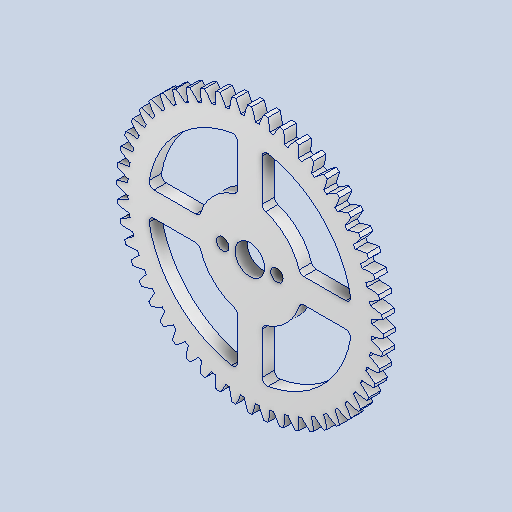
# Autodesk Inventor part: 平歯車1
Saved by Autodesk Inventor 2025.2 (Build 292293000, 293)
## iProperties
CustomPartVersion: 1
Created: 2025-05-14
Part Number: 平歯車1
Material: アルミニウム 6061
Document SubType Name: Modeling
Designer: haruy
Categories: <?xml version="1.0" encoding="UTF-16"?> <MemberInstance><Categories><FamilyTemplate><FamilyTemplateParameter ValueType="xs:double" Id="1" ObjectReferenceKey="da_z" ObjectType="kUserParameterObject"/><FamilyTemplateParameter ValueType="xs:double" Id="2" ObjectReferenceKey="da_b" ObjectType="kUserParameterObject"/><FamilyTemplateParameter ValueType="xs:double" Id="3" ObjectReferenceKey="da_beta" ObjectType="kUserParameterObject"/><FamilyTemplateParameter ValueType="xs:double" Id="4" ObjectReferenceKey="da_da" ObjectType="kUserParameterObject"/><FamilyTemplateParameter ValueType="xs:double" Id="5" ObjectReferenceKey="da_aw" ObjectType="kUserParameterObject"/><FamilyTemplateParameter ValueType="xs:string" Id="6" ObjectReferenceKey="EAIAABAAAACIAQAAAAAAAIAAAAAAAAAA" ObjectType="83910656" SubObjectId="SurfaceGeometry"/></FamilyTemplate><ParamToTemplateMap><ParamToTemplate CategoryParameter="//CategoryParameter[@InternalName='046C89C9-8512-4d59-83FE-43B91F4F132A']" TemplateParameter="1"/><ParamToTemplate CategoryParameter="//CategoryParameter[@InternalName='2552DF32-E462-4b46-AEBF-C6C7768E72AC']" TemplateParameter="2"/><ParamToTemplate CategoryParameter="//CategoryParameter[@InternalName='C9EE641D-15FC-4fae-A226-E94C4372FDD7']" TemplateParameter="3"/><ParamToTemplate><ParamToTemplate CategoryParameter="//CategoryParameter[@InternalName='00B6519A-459B-49c7-AD84-2E56D39A5744']" ConstantValue="0.000000"/></ParamToTemplate><ParamToTemplate><ParamToTemplate CategoryParameter="//CategoryParameter[@InternalName='04B31F0E-C7A6-4894-AA32-9629BEFACF47']" ConstantValue="1.000000"/></ParamToTemplate><ParamToTemplate><ParamToTemplate CategoryParameter="//CategoryParameter[@InternalName='43CBEC2E-7847-49e7-A936-2F7889FCB2D9']" ConstantValue="0.250000"/></ParamToTemplate><ParamToTemplate><ParamToTemplate CategoryParameter="//CategoryParameter[@InternalName='B1EFC894-105D-4ebd-86BF-FA20ED196853']" ConstantValue="0.350000"/></ParamToTemplate><ParamToTemplate><ParamToTemplate CategoryParameter="//CategoryParameter[@InternalName='51175063-3D10-4879-93E8-6246FE8B403D']" ConstantValue="2060000000.000000"/></ParamToTemplate><ParamToTemplate><ParamToTemplate CategoryParameter="//CategoryParameter[@InternalName='A3A52E27-4454-46a9-B0BD-C932399B70AF']" ConstantValue="0.300000"/></ParamToTemplate><ParamToTemplate><ParamToTemplate CategoryParameter="//CategoryParameter[@InternalName='91B76062-C214-41d9-B1B9-14D2AB99603D']" ConstantValue="0.200000"/></ParamToTemplate><ParamToTemplate><ParamToTemplate CategoryParameter="//CategoryParameter[@InternalName='374E806E-8B8A-4dda-A9AA-1039D6500AD2']" ConstantValue="5.000000"/></ParamToTemplate><ParamToTemplate><ParamToTemplate CategoryParameter="//CategoryParameter[@InternalName='2D373A89-B862-43d6-8D0B-0CBF12AB9F6C']" ConstantValue="0.349066"/></ParamToTemplate><ParamToTemplate CategoryParameter="//CategoryParameter[@InternalName='37777632-D6A2-4fac-9D53-DB8ACD95C989']" TemplateParameter="4"/><ParamToTemplate CategoryParameter="//CategoryParameter[@InternalName='FD1017F1-B727-4f7e-9707-0F86F1FF9423']" TemplateParameter="5"/><ParamToTemplate><ParamToTemplate CategoryParameter="//CategoryParameter[@InternalName='9E1B4470-B2D3-4ff1-B813-535BB4CDF51A']" ConstantValue="3520000.000000"/></ParamToTemplate><ParamToTemplate><ParamToTemplate CategoryParameter="//CategoryParameter[@InternalName='F8452263-BFF6-458c-9FB1-07C4B99E95CD']" ConstantValue="11400000.000000"/></ParamToTemplate><ParamToTemplate><ParamToTemplate CategoryParameter="//CategoryParameter[@InternalName='3E3BB259-FD49-497f-8171-6EBC954A3479']" ConstantValue="2.000000"/></ParamToTemplate><ParamToTemplate CategoryParameter="//CategoryParameter[@InternalName='27C3BAF2-7550-4e4b-AE2C-0DB134B7D9B7']" TemplateParameter="6"/></ParamToTemplateMap><Category DisplayName="Gear" InternalName="DC85795E-93AB-48d5-8EEE-5A27447B64BD" Mnemonic="Gear"><CategoryParameter DisplayName="z" InternalName="046C89C9-8512-4d59-83FE-43B91F4F132A" Mnemonic="z"/><CategoryParameter DisplayName="b" InternalName="2552DF32-E462-4b46-AEBF-C6C7768E72AC" Mnemonic="b"/><CategoryParameter DisplayName="||b|" InternalName="C9EE641D-15FC-4fae-A226-E94C4372FDD7" Mnemonic="beta"/><CategoryParameter DisplayName="x" InternalName="00B6519A-459B-49c7-AD84-2E56D39A5744" Mnemonic="x"/><CategoryParameter DisplayName="a*" InternalName="04B31F0E-C7A6-4894-AA32-9629BEFACF47" Mnemonic="a"/><CategoryParameter DisplayName="c*" InternalName="43CBEC2E-7847-49e7-A936-2F7889FCB2D9" Mnemonic="c"/><CategoryParameter DisplayName="r|.f|*" InternalName="B1EFC894-105D-4ebd-86BF-FA20ED196853" Mnemonic="rf"/><CategoryParameter DisplayName="E" InternalName="51175063-3D10-4879-93E8-6246FE8B403D" Mnemonic="E"/><CategoryParameter DisplayName="||m|" InternalName="A3A52E27-4454-46a9-B0BD-C932399B70AF" Mnemonic="mi"/><Category DisplayName="SpurGear" InternalName="26C5A22E-A91E-4dfd-A3B3-23CCAFAE1764" Mnemonic="SpurGear"><CategoryParameter DisplayName="m" InternalName="91B76062-C214-41d9-B1B9-14D2AB99603D" Mnemonic="m"/><CategoryParameter DisplayName="P" InternalName="374E806E-8B8A-4dda-A9AA-1039D6500AD2" Mnemonic="PP"/><CategoryParameter DisplayName="||a|" InternalName="2D373A89-B862-43d6-8D0B-0CBF12AB9F6C" Mnemonic="alpha"/><CategoryParameter DisplayName="d|.a|" InternalName="37777632-D6A2-4fac-9D53-DB8ACD95C989" Mnemonic="da"/><CategoryParameter DisplayName="a|.w|" InternalName="FD1017F1-B727-4f7e-9707-0F86F1FF9423" Mnemonic="aw"/><CategoryParameter DisplayName="||s||.Flim|" InternalName="9E1B4470-B2D3-4ff1-B813-535BB4CDF51A" Mnemonic="sFlim"/><CategoryParameter DisplayName="||s||.Hlim|" InternalName="F8452263-BFF6-458c-9FB1-07C4B99E95CD" Mnemonic="sHlim"/><CategoryParameter DisplayName="タイプ" InternalName="3E3BB259-FD49-497f-8171-6EBC954A3479" Mnemonic="type"/><CategoryParameter DisplayName="PitchDiameter" InternalName="27C3BAF2-7550-4e4b-AE2C-0DB134B7D9B7" Mnemonic="IDS_PITCHDIAM"/></Category></Category></Categories></MemberInstance>
Density: 2.7 g/cm^3
Appearance: アルミニウム - フラット
Author: haruy
Autodesk Inventor part; units mm, degrees
sketch "Sketch1" plane through (0, 0, 0) normal (0, 0, 1) x (1, 0, 0)
  circle A0 centre (0, 0) radius 54
  dimension "d0" = 108
  constraints: 1 centre point
  measures "d0" diameter of A0
extrude "Extrusion1" add sketch "Sketch1" along normal blind 5
ref_plane "Work Plane2" through (0, 0, 2.5) normal (0, 0, 1) x (1, 0, 0)
sketch "Sketch2" plane through (0, 0, 0) normal (0, 0, -1) x (-1, 0, 0)
  circle A0 centre (0, 0) radius 54 projected
  circle A1 centre (0, 0) radius 52
  dimension "d3" = 104
  constraints: 1 centre point, 1 coincident
  measures "d3" diameter of A1
surface extrude "ピッチ円直径" sketch "Sketch2" against normal through all shown no curves A1
ref_plane "Work Plane8" through (0, 0, 0) normal (0.9981756, 0.0603785, 0) x (0, 0, 1)
ref_plane "Work Plane9" through (0, 0, 0) normal (1, 0, 0) x (0, 1, 0)
spur gear teeth "平歯車" teeth 52 pitch diameter 104 tip diameter 108 root diameter 99 face width 5 start plane through (0, 0, 0) normal (0, 0, -1) x (-1, 0, 0)
sketch "スケッチ3" plane through (0, 0, 5) normal (0, 0, 1) x (1, 0, 0)
  circle A0 centre (0, 0) radius 6
  circle A1 centre (0, 0) radius 11
  circle A2 centre (-11, 0) radius 2.5
  circle A3 centre (11, 0) radius 2.5
  circle A4 centre (0, 0) radius 49.5
  circle A5 centre (0, 0) radius 21
  circle A6 centre (0, 0) radius 41.5
  line L0 (-5, 41.1977) -> (-5, 20.3961)
  line L1 (0, 0) -> (0, 49.5)
  line L2 (5, 41.1977) -> (5, 20.3961)
  line L3 (-41.1977, -5) -> (-20.3961, -5)
  line L4 (-41.1977, 5) -> (-20.3961, 5)
  line L5 (5, -41.1977) -> (5, -20.3961)
  line L6 (-5, -41.1977) -> (-5, -20.3961)
  line L7 (41.1977, 5) -> (20.3961, 5)
  line L8 (41.1977, -5) -> (20.3961, -5)
  point P0 (-49.4492, 2.2421)
  dimension "d50" = 22
  dimension "d56" = 10
  dimension "d49" = 12
  dimension "d51" = 5
  dimension "d54" = 360
  dimension "d57" = 8
  dimension "d58" = 5
  dimension "d61" = 360
  constraints: 18 end point, 4 centre point, 3 coincident, 2 point on circle, 2 symmetric about line, 1 horizontal alignment, 1 parallel, 1 vertical, 38 other
  measures "d49" diameter of A0
  measures "d51" diameter of A2
  measures "d58" distance between parallel lines of L1 L0
extrude "押し出し2" cut sketch "スケッチ3" against normal blind 10 contours A0 | A1 A3 | A1 A3 | A2 A1 | A1 A2 | A5 L2 A6 L7 | L8 A6 L5 A5 | L6 A6 L3 A5 | A5 L4 A6 L0
fillet "フィレット1" radius 2 16 edges at (-41.1977, -5, 2.5) (-20.3961, -5, 2.5) (-5, -20.3961, 2.5) (-5, -41.1977, 2.5) (5, -20.3961, 2.5) (5, -41.1977, 2.5) (41.1977, -5, 2.5) (20.3961, -5, 2.5) (20.3961, 5, 2.5) (41.1977, 5, 2.5) (5, 20.3961, 2.5) (5, 41.1977, 2.5) (-5, 41.1977, 2.5) (-5, 20.3961, 2.5) (-20.3961, 5, 2.5) (-41.1977, 5, 2.5)
sketch "スケッチ5" plane through (0, 0, 5) normal (0, 0, 1) x (1, 0, 0)
  line L0 (5, -38.8748) -> (5, -21.9089) projected
  arc A0 (6.3913, -20.0038) -> (5, -21.9089) centre (7, -21.9089) ccw projected
  arc A1 (6.3913, -20.0038) -> (20.0038, -6.3913) centre (0, 0) ccw projected
  arc A2 (21.9089, -5) -> (20.0038, -6.3913) centre (21.9089, -7) ccw projected
  line L1 (21.9089, -5) -> (38.8748, -5) projected
  arc A3 (40.8431, -7.3544) -> (38.8748, -5) centre (38.8748, -7) ccw projected
  arc A4 (7.3544, -40.8431) -> (40.8431, -7.3544) centre (0, 0) ccw projected
  arc A5 (5, -38.8748) -> (7.3544, -40.8431) centre (7, -38.8748) ccw projected
  circle A6 centre (11, 0) radius 2.5 projected
  line L2 (5, 21.9089) -> (5, 38.8748) projected
  arc A7 (7.3544, 40.8431) -> (5, 38.8748) centre (7, 38.8748) ccw projected
  arc A8 (40.8431, 7.3544) -> (7.3544, 40.8431) centre (0, 0) ccw projected
  arc A9 (38.8748, 5) -> (40.8431, 7.3544) centre (38.8748, 7) ccw projected
  line L3 (38.8748, 5) -> (21.9089, 5) projected
  arc A10 (20.0038, 6.3913) -> (21.9089, 5) centre (21.9089, 7) ccw projected
  arc A11 (20.0038, 6.3913) -> (6.3913, 20.0038) centre (0, 0) ccw projected
  arc A12 (5, 21.9089) -> (6.3913, 20.0038) centre (7, 21.9089) ccw projected
  line L4 (-38.8748, -5) -> (-21.9089, -5) projected
  arc A13 (-20.0038, -6.3913) -> (-21.9089, -5) centre (-21.9089, -7) ccw projected
  arc A14 (-20.0038, -6.3913) -> (-6.3913, -20.0038) centre (0, 0) ccw projected
  arc A15 (-5, -21.9089) -> (-6.3913, -20.0038) centre (-7, -21.9089) ccw projected
  line L5 (-5, -21.9089) -> (-5, -38.8748) projected
  arc A16 (-7.3544, -40.8431) -> (-5, -38.8748) centre (-7, -38.8748) ccw projected
  arc A17 (-40.8431, -7.3544) -> (-7.3544, -40.8431) centre (0, 0) ccw projected
  arc A18 (-38.8748, -5) -> (-40.8431, -7.3544) centre (-38.8748, -7) ccw projected
  circle A19 centre (-11, 0) radius 2.5 projected
  circle A20 centre (0, 0) radius 6 projected
  line L6 (-5, 38.8748) -> (-5, 21.9089) projected
  arc A21 (-6.3913, 20.0038) -> (-5, 21.9089) centre (-7, 21.9089) ccw projected
  arc A22 (-6.3913, 20.0038) -> (-20.0038, 6.3913) centre (0, 0) ccw projected
  arc A23 (-21.9089, 5) -> (-20.0038, 6.3913) centre (-21.9089, 7) ccw projected
  line L7 (-21.9089, 5) -> (-38.8748, 5) projected
  arc A24 (-40.8431, 7.3544) -> (-38.8748, 5) centre (-38.8748, 7) ccw projected
  arc A25 (-7.3544, 40.8431) -> (-40.8431, 7.3544) centre (0, 0) ccw projected
  arc A26 (-5, 38.8748) -> (-7.3544, 40.8431) centre (-7, 38.8748) ccw projected
  arc A27 (-7.3179, 53.5019) -> (-8.1862, 48.8184) centre (15.9886, 46.7583) ccw projected
  arc A28 (-8.1862, 48.8184) -> (-9.657, 48.5489) centre (0, 0) ccw projected
  arc A29 (-9.657, 48.5489) -> (-12.1297, 52.6201) centre (-31.5303, 38.0502) ccw projected
  arc A30 (-12.1297, 52.6201) -> (-13.7134, 52.2297) centre (0, 0) ccw projected
  arc A31 (-13.7134, 52.2297) -> (-14.011, 47.4757) centre (10.2359, 48.3446) ccw projected
  arc A32 (-14.011, 47.4757) -> (-15.4385, 47.0309) centre (0, 0) ccw projected
  arc A33 (-15.4385, 47.0309) -> (-18.3839, 50.7743) centre (-35.8868, 33.9722) ccw projected
  arc A34 (-18.3839, 50.7743) -> (-19.9091, 50.1959) centre (0, 0) ccw projected
  arc A35 (-19.9091, 50.1959) -> (-19.6314, 45.4407) centre (4.334, 49.2259) ccw projected
  arc A36 (-19.6314, 45.4407) -> (-20.9949, 44.8271) centre (0, 0) ccw projected
  arc A37 (-20.9949, 44.8271) -> (-24.37, 48.1882) centre (-39.7201, 29.3988) ccw projected
  arc A38 (-24.37, 48.1882) -> (-25.8143, 47.4302) centre (0, 0) ccw projected
  arc A39 (-25.8143, 47.4302) -> (-24.9655, 42.7431) centre (-1.6312, 49.3894) ccw projected
  arc A40 (-24.9655, 42.7431) -> (-26.2451, 41.9696) centre (0, 0) ccw projected
  arc A41 (-26.2451, 41.9696) -> (-30.0008, 44.8994) centre (-42.9741, 24.3967) ccw projected
  arc A42 (-30.0008, 44.8994) -> (-31.3432, 43.9728) centre (0, 0) ccw projected
  arc A43 (-31.3432, 43.9728) -> (-29.9356, 39.4222) centre (-7.5725, 48.8327) ccw projected
  arc A44 (-29.9356, 39.4222) -> (-31.1126, 38.5001) centre (0, 0) ccw projected
  arc A45 (-31.1126, 38.5001) -> (-35.1941, 40.9558) centre (-45.6015, 19.0389) ccw projected
  arc A46 (-35.1941, 40.9558) -> (-36.415, 39.8741) centre (0, 0) ccw projected
  arc A47 (-36.415, 39.8741) -> (-34.4692, 35.5264) centre (-13.4034, 47.5639) ccw projected
  arc A48 (-34.4692, 35.5264) -> (-35.5264, 34.4692) centre (0, 0) ccw projected
  arc A49 (-35.5264, 34.4692) -> (-39.8741, 36.415) centre (-47.5639, 13.4034) ccw projected
  arc A50 (-39.8741, 36.415) -> (-40.9558, 35.1941) centre (0, 0) ccw projected
  arc A51 (-40.9558, 35.1941) -> (-38.5001, 31.1126) centre (-19.0389, 45.6015) ccw projected
  arc A52 (-38.5001, 31.1126) -> (-39.4222, 29.9356) centre (0, 0) ccw projected
  arc A53 (-39.4222, 29.9356) -> (-43.9728, 31.3432) centre (-48.8327, 7.5725) ccw projected
  arc A54 (-43.9728, 31.3432) -> (-44.8994, 30.0008) centre (0, 0) ccw projected
  arc A55 (-44.8994, 30.0008) -> (-41.9696, 26.2451) centre (-24.3967, 42.9741) ccw projected
  arc A56 (-41.9696, 26.2451) -> (-42.7431, 24.9655) centre (0, 0) ccw projected
  arc A57 (-42.7431, 24.9655) -> (-47.4302, 25.8143) centre (-49.3894, 1.6312) ccw projected
  arc A58 (-47.4302, 25.8143) -> (-48.1882, 24.37) centre (0, 0) ccw projected
  arc A59 (-48.1882, 24.37) -> (-44.8271, 20.9949) centre (-29.3988, 39.7201) ccw projected
  arc A60 (-44.8271, 20.9949) -> (-45.4407, 19.6314) centre (0, 0) ccw projected
  arc A61 (-45.4407, 19.6314) -> (-50.1959, 19.9091) centre (-49.2259, -4.334) ccw projected
  arc A62 (-50.1959, 19.9091) -> (-50.7743, 18.3839) centre (0, 0) ccw projected
  arc A63 (-50.7743, 18.3839) -> (-47.0309, 15.4385) centre (-33.9722, 35.8868) ccw projected
  arc A64 (-47.0309, 15.4385) -> (-47.4757, 14.011) centre (0, 0) ccw projected
  arc A65 (-47.4757, 14.011) -> (-52.2297, 13.7134) centre (-48.3446, -10.2359) ccw projected
  arc A66 (-52.2297, 13.7134) -> (-52.6201, 12.1297) centre (0, 0) ccw projected
  arc A67 (-52.6201, 12.1297) -> (-48.5489, 9.657) centre (-38.0502, 31.5303) ccw projected
  arc A68 (-48.5489, 9.657) -> (-48.8184, 8.1862) centre (0, 0) ccw projected
  arc A69 (-48.8184, 8.1862) -> (-53.5019, 7.3179) centre (-46.7583, -15.9886) ccw projected
  arc A70 (-53.5019, 7.3179) -> (-53.6985, 5.6986) centre (0, 0) ccw projected
  arc A71 (-53.6985, 5.6986) -> (-49.3589, 3.7346) centre (-41.5733, 26.7139) ccw projected
  arc A72 (-49.3589, 3.7346) -> (-49.4492, 2.2421) centre (0, 0) ccw projected
  arc A73 (-49.4492, 2.2421) -> (-53.9938, 0.8156) centre (-44.4902, -21.5081) ccw projected
  arc A74 (-53.9938, 0.8156) -> (-53.9938, -0.8156) centre (0, 0) ccw projected
  arc A75 (-53.9938, -0.8156) -> (-49.4492, -2.2421) centre (-44.4902, 21.5081) ccw projected
  arc A76 (-49.4492, -2.2421) -> (-49.3589, -3.7346) centre (0, 0) ccw projected
  arc A77 (-49.3589, -3.7346) -> (-53.6985, -5.6986) centre (-41.5733, -26.7139) ccw projected
  arc A78 (-53.6985, -5.6986) -> (-53.5019, -7.3179) centre (0, 0) ccw projected
  arc A79 (-53.5019, -7.3179) -> (-48.8184, -8.1862) centre (-46.7583, 15.9886) ccw projected
  arc A80 (-48.8184, -8.1862) -> (-48.5489, -9.657) centre (0, 0) ccw projected
  arc A81 (-48.5489, -9.657) -> (-52.6201, -12.1297) centre (-38.0502, -31.5303) ccw projected
  arc A82 (-52.6201, -12.1297) -> (-52.2297, -13.7134) centre (0, 0) ccw projected
  arc A83 (-52.2297, -13.7134) -> (-47.4757, -14.011) centre (-48.3446, 10.2359) ccw projected
  arc A84 (-47.4757, -14.011) -> (-47.0309, -15.4385) centre (0, 0) ccw projected
  arc A85 (-47.0309, -15.4385) -> (-50.7743, -18.3839) centre (-33.9722, -35.8868) ccw projected
  arc A86 (-50.7743, -18.3839) -> (-50.1959, -19.9091) centre (0, 0) ccw projected
  arc A87 (-50.1959, -19.9091) -> (-45.4407, -19.6314) centre (-49.2259, 4.334) ccw projected
  arc A88 (-45.4407, -19.6314) -> (-44.8271, -20.9949) centre (0, 0) ccw projected
  arc A89 (-44.8271, -20.9949) -> (-48.1882, -24.37) centre (-29.3988, -39.7201) ccw projected
  arc A90 (-48.1882, -24.37) -> (-47.4302, -25.8143) centre (0, 0) ccw projected
  arc A91 (-47.4302, -25.8143) -> (-42.7431, -24.9655) centre (-49.3894, -1.6312) ccw projected
  arc A92 (-42.7431, -24.9655) -> (-41.9696, -26.2451) centre (0, 0) ccw projected
  arc A93 (-41.9696, -26.2451) -> (-44.8994, -30.0008) centre (-24.3967, -42.9741) ccw projected
  arc A94 (-44.8994, -30.0008) -> (-43.9728, -31.3432) centre (0, 0) ccw projected
  arc A95 (-43.9728, -31.3432) -> (-39.4222, -29.9356) centre (-48.8327, -7.5725) ccw projected
  arc A96 (-39.4222, -29.9356) -> (-38.5001, -31.1126) centre (0, 0) ccw projected
  arc A97 (-38.5001, -31.1126) -> (-40.9558, -35.1941) centre (-19.0389, -45.6015) ccw projected
  arc A98 (-40.9558, -35.1941) -> (-39.8741, -36.415) centre (0, 0) ccw projected
  arc A99 (-39.8741, -36.415) -> (-35.5264, -34.4692) centre (-47.5639, -13.4034) ccw projected
  arc A100 (-35.5264, -34.4692) -> (-34.4692, -35.5264) centre (0, 0) ccw projected
  arc A101 (-34.4692, -35.5264) -> (-36.415, -39.8741) centre (-13.4034, -47.5639) ccw projected
  arc A102 (-36.415, -39.8741) -> (-35.1941, -40.9558) centre (0, 0) ccw projected
  arc A103 (-35.1941, -40.9558) -> (-31.1126, -38.5001) centre (-45.6015, -19.0389) ccw projected
  arc A104 (-31.1126, -38.5001) -> (-29.9356, -39.4222) centre (0, 0) ccw projected
  arc A105 (-29.9356, -39.4222) -> (-31.3432, -43.9728) centre (-7.5725, -48.8327) ccw projected
  arc A106 (-31.3432, -43.9728) -> (-30.0008, -44.8994) centre (0, 0) ccw projected
  arc A107 (-30.0008, -44.8994) -> (-26.2451, -41.9696) centre (-42.9741, -24.3967) ccw projected
  arc A108 (-26.2451, -41.9696) -> (-24.9655, -42.7431) centre (0, 0) ccw projected
  arc A109 (-24.9655, -42.7431) -> (-25.8143, -47.4302) centre (-1.6312, -49.3894) ccw projected
  arc A110 (-25.8143, -47.4302) -> (-24.37, -48.1882) centre (0, 0) ccw projected
  arc A111 (-24.37, -48.1882) -> (-20.9949, -44.8271) centre (-39.7201, -29.3988) ccw projected
  arc A112 (-20.9949, -44.8271) -> (-19.6314, -45.4407) centre (0, 0) ccw projected
  arc A113 (-19.6314, -45.4407) -> (-19.9091, -50.1959) centre (4.334, -49.2259) ccw projected
  arc A114 (-19.9091, -50.1959) -> (-18.3839, -50.7743) centre (0, 0) ccw projected
  arc A115 (-18.3839, -50.7743) -> (-15.4385, -47.0309) centre (-35.8868, -33.9722) ccw projected
  arc A116 (-15.4385, -47.0309) -> (-14.011, -47.4757) centre (0, 0) ccw projected
  arc A117 (-14.011, -47.4757) -> (-13.7134, -52.2297) centre (10.2359, -48.3446) ccw projected
  arc A118 (-13.7134, -52.2297) -> (-12.1297, -52.6201) centre (0, 0) ccw projected
  arc A119 (-12.1297, -52.6201) -> (-9.657, -48.5489) centre (-31.5303, -38.0502) ccw projected
  arc A120 (-9.657, -48.5489) -> (-8.1862, -48.8184) centre (0, 0) ccw projected
  arc A121 (-8.1862, -48.8184) -> (-7.3179, -53.5019) centre (15.9886, -46.7583) ccw projected
  arc A122 (-7.3179, -53.5019) -> (-5.6986, -53.6985) centre (0, 0) ccw projected
  arc A123 (-5.6986, -53.6985) -> (-3.7346, -49.3589) centre (-26.7139, -41.5733) ccw projected
  arc A124 (-3.7346, -49.3589) -> (-2.2421, -49.4492) centre (0, 0) ccw projected
  arc A125 (-2.2421, -49.4492) -> (-0.8156, -53.9938) centre (21.5081, -44.4902) ccw projected
  arc A126 (-0.8156, -53.9938) -> (0.8156, -53.9938) centre (0, 0) ccw projected
  arc A127 (0.8156, -53.9938) -> (2.2421, -49.4492) centre (-21.5081, -44.4902) ccw projected
  arc A128 (2.2421, -49.4492) -> (3.7346, -49.3589) centre (0, 0) ccw projected
  arc A129 (3.7346, -49.3589) -> (5.6986, -53.6985) centre (26.7139, -41.5733) ccw projected
  arc A130 (5.6986, -53.6985) -> (7.3179, -53.5019) centre (0, 0) ccw projected
  arc A131 (7.3179, -53.5019) -> (8.1862, -48.8184) centre (-15.9886, -46.7583) ccw projected
  arc A132 (8.1862, -48.8184) -> (9.657, -48.5489) centre (0, 0) ccw projected
  arc A133 (9.657, -48.5489) -> (12.1297, -52.6201) centre (31.5303, -38.0502) ccw projected
  arc A134 (12.1297, -52.6201) -> (13.7134, -52.2297) centre (0, 0) ccw projected
  arc A135 (13.7134, -52.2297) -> (14.011, -47.4757) centre (-10.2359, -48.3446) ccw projected
  arc A136 (14.011, -47.4757) -> (15.4385, -47.0309) centre (0, 0) ccw projected
  arc A137 (15.4385, -47.0309) -> (18.3839, -50.7743) centre (35.8868, -33.9722) ccw projected
  arc A138 (18.3839, -50.7743) -> (19.9091, -50.1959) centre (0, 0) ccw projected
  arc A139 (19.9091, -50.1959) -> (19.6314, -45.4407) centre (-4.334, -49.2259) ccw projected
  arc A140 (19.6314, -45.4407) -> (20.9949, -44.8271) centre (0, 0) ccw projected
  arc A141 (20.9949, -44.8271) -> (24.37, -48.1882) centre (39.7201, -29.3988) ccw projected
  arc A142 (24.37, -48.1882) -> (25.8143, -47.4302) centre (0, 0) ccw projected
  arc A143 (25.8143, -47.4302) -> (24.9655, -42.7431) centre (1.6312, -49.3894) ccw projected
  arc A144 (24.9655, -42.7431) -> (26.2451, -41.9696) centre (0, 0) ccw projected
  arc A145 (26.2451, -41.9696) -> (30.0008, -44.8994) centre (42.9741, -24.3967) ccw projected
  arc A146 (30.0008, -44.8994) -> (31.3432, -43.9728) centre (0, 0) ccw projected
  arc A147 (31.3432, -43.9728) -> (29.9356, -39.4222) centre (7.5725, -48.8327) ccw projected
  arc A148 (29.9356, -39.4222) -> (31.1126, -38.5001) centre (0, 0) ccw projected
  arc A149 (31.1126, -38.5001) -> (35.1941, -40.9558) centre (45.6015, -19.0389) ccw projected
  arc A150 (35.1941, -40.9558) -> (36.415, -39.8741) centre (0, 0) ccw projected
  arc A151 (36.415, -39.8741) -> (34.4692, -35.5264) centre (13.4034, -47.5639) ccw projected
  arc A152 (34.4692, -35.5264) -> (35.5264, -34.4692) centre (0, 0) ccw projected
  arc A153 (35.5264, -34.4692) -> (39.8741, -36.415) centre (47.5639, -13.4034) ccw projected
  arc A154 (39.8741, -36.415) -> (40.9558, -35.1941) centre (0, 0) ccw projected
  arc A155 (40.9558, -35.1941) -> (38.5001, -31.1126) centre (19.0389, -45.6015) ccw projected
  arc A156 (38.5001, -31.1126) -> (39.4222, -29.9356) centre (0, 0) ccw projected
  arc A157 (39.4222, -29.9356) -> (43.9728, -31.3432) centre (48.8327, -7.5725) ccw projected
  arc A158 (43.9728, -31.3432) -> (44.8994, -30.0008) centre (0, 0) ccw projected
  arc A159 (44.8994, -30.0008) -> (41.9696, -26.2451) centre (24.3967, -42.9741) ccw projected
  arc A160 (41.9696, -26.2451) -> (42.7431, -24.9655) centre (0, 0) ccw projected
  arc A161 (42.7431, -24.9655) -> (47.4302, -25.8143) centre (49.3894, -1.6312) ccw projected
  arc A162 (47.4302, -25.8143) -> (48.1882, -24.37) centre (0, 0) ccw projected
  arc A163 (48.1882, -24.37) -> (44.8271, -20.9949) centre (29.3988, -39.7201) ccw projected
  arc A164 (44.8271, -20.9949) -> (45.4407, -19.6314) centre (0, 0) ccw projected
  arc A165 (45.4407, -19.6314) -> (50.1959, -19.9091) centre (49.2259, 4.334) ccw projected
  arc A166 (50.1959, -19.9091) -> (50.7743, -18.3839) centre (0, 0) ccw projected
  arc A167 (50.7743, -18.3839) -> (47.0309, -15.4385) centre (33.9722, -35.8868) ccw projected
  arc A168 (47.0309, -15.4385) -> (47.4757, -14.011) centre (0, 0) ccw projected
  arc A169 (47.4757, -14.011) -> (52.2297, -13.7134) centre (48.3446, 10.2359) ccw projected
  arc A170 (52.2297, -13.7134) -> (52.6201, -12.1297) centre (0, 0) ccw projected
  arc A171 (52.6201, -12.1297) -> (48.5489, -9.657) centre (38.0502, -31.5303) ccw projected
  arc A172 (48.5489, -9.657) -> (48.8184, -8.1862) centre (0, 0) ccw projected
  arc A173 (48.8184, -8.1862) -> (53.5019, -7.3179) centre (46.7583, 15.9886) ccw projected
  arc A174 (53.5019, -7.3179) -> (53.6985, -5.6986) centre (0, 0) ccw projected
  arc A175 (53.6985, -5.6986) -> (49.3589, -3.7346) centre (41.5733, -26.7139) ccw projected
  arc A176 (49.3589, -3.7346) -> (49.4492, -2.2421) centre (0, 0) ccw projected
  arc A177 (49.4492, -2.2421) -> (53.9938, -0.8156) centre (44.4902, 21.5081) ccw projected
  arc A178 (53.9938, -0.8156) -> (53.9938, 0.8156) centre (0, 0) ccw projected
  arc A179 (53.9938, 0.8156) -> (49.4492, 2.2421) centre (44.4902, -21.5081) ccw projected
  arc A180 (49.4492, 2.2421) -> (49.3589, 3.7346) centre (0, 0) ccw projected
  arc A181 (49.3589, 3.7346) -> (53.6985, 5.6986) centre (41.5733, 26.7139) ccw projected
  arc A182 (53.6985, 5.6986) -> (53.5019, 7.3179) centre (0, 0) ccw projected
  arc A183 (53.5019, 7.3179) -> (48.8184, 8.1862) centre (46.7583, -15.9886) ccw projected
  arc A184 (48.8184, 8.1862) -> (48.5489, 9.657) centre (0, 0) ccw projected
  arc A185 (48.5489, 9.657) -> (52.6201, 12.1297) centre (38.0502, 31.5303) ccw projected
  arc A186 (52.6201, 12.1297) -> (52.2297, 13.7134) centre (0, 0) ccw projected
  arc A187 (52.2297, 13.7134) -> (47.4757, 14.011) centre (48.3446, -10.2359) ccw projected
  arc A188 (47.4757, 14.011) -> (47.0309, 15.4385) centre (0, 0) ccw projected
  arc A189 (47.0309, 15.4385) -> (50.7743, 18.3839) centre (33.9722, 35.8868) ccw projected
  arc A190 (50.7743, 18.3839) -> (50.1959, 19.9091) centre (0, 0) ccw projected
  arc A191 (50.1959, 19.9091) -> (45.4407, 19.6314) centre (49.2259, -4.334) ccw projected
  arc A192 (45.4407, 19.6314) -> (44.8271, 20.9949) centre (0, 0) ccw projected
  arc A193 (44.8271, 20.9949) -> (48.1882, 24.37) centre (29.3988, 39.7201) ccw projected
  arc A194 (48.1882, 24.37) -> (47.4302, 25.8143) centre (0, 0) ccw projected
  arc A195 (47.4302, 25.8143) -> (42.7431, 24.9655) centre (49.3894, 1.6312) ccw projected
  arc A196 (42.7431, 24.9655) -> (41.9696, 26.2451) centre (0, 0) ccw projected
  arc A197 (41.9696, 26.2451) -> (44.8994, 30.0008) centre (24.3967, 42.9741) ccw projected
  arc A198 (44.8994, 30.0008) -> (43.9728, 31.3432) centre (0, 0) ccw projected
  arc A199 (43.9728, 31.3432) -> (39.4222, 29.9356) centre (48.8327, 7.5725) ccw projected
  arc A200 (39.4222, 29.9356) -> (38.5001, 31.1126) centre (0, 0) ccw projected
  arc A201 (38.5001, 31.1126) -> (40.9558, 35.1941) centre (19.0389, 45.6015) ccw projected
  arc A202 (40.9558, 35.1941) -> (39.8741, 36.415) centre (0, 0) ccw projected
  arc A203 (39.8741, 36.415) -> (35.5264, 34.4692) centre (47.5639, 13.4034) ccw projected
  arc A204 (35.5264, 34.4692) -> (34.4692, 35.5264) centre (0, 0) ccw projected
  arc A205 (34.4692, 35.5264) -> (36.415, 39.8741) centre (13.4034, 47.5639) ccw projected
  arc A206 (36.415, 39.8741) -> (35.1941, 40.9558) centre (0, 0) ccw projected
  arc A207 (35.1941, 40.9558) -> (31.1126, 38.5001) centre (45.6015, 19.0389) ccw projected
  arc A208 (31.1126, 38.5001) -> (29.9356, 39.4222) centre (0, 0) ccw projected
  arc A209 (29.9356, 39.4222) -> (31.3432, 43.9728) centre (7.5725, 48.8327) ccw projected
  arc A210 (31.3432, 43.9728) -> (30.0008, 44.8994) centre (0, 0) ccw projected
  arc A211 (30.0008, 44.8994) -> (26.2451, 41.9696) centre (42.9741, 24.3967) ccw projected
  arc A212 (26.2451, 41.9696) -> (24.9655, 42.7431) centre (0, 0) ccw projected
  arc A213 (24.9655, 42.7431) -> (25.8143, 47.4302) centre (1.6312, 49.3894) ccw projected
  arc A214 (25.8143, 47.4302) -> (24.37, 48.1882) centre (0, 0) ccw projected
  arc A215 (24.37, 48.1882) -> (20.9949, 44.8271) centre (39.7201, 29.3988) ccw projected
  arc A216 (20.9949, 44.8271) -> (19.6314, 45.4407) centre (0, 0) ccw projected
  arc A217 (19.6314, 45.4407) -> (19.9091, 50.1959) centre (-4.334, 49.2259) ccw projected
  arc A218 (19.9091, 50.1959) -> (18.3839, 50.7743) centre (0, 0) ccw projected
  arc A219 (18.3839, 50.7743) -> (15.4385, 47.0309) centre (35.8868, 33.9722) ccw projected
  arc A220 (15.4385, 47.0309) -> (14.011, 47.4757) centre (0, 0) ccw projected
  arc A221 (14.011, 47.4757) -> (13.7134, 52.2297) centre (-10.2359, 48.3446) ccw projected
  arc A222 (13.7134, 52.2297) -> (12.1297, 52.6201) centre (0, 0) ccw projected
  arc A223 (12.1297, 52.6201) -> (9.657, 48.5489) centre (31.5303, 38.0502) ccw projected
  arc A224 (9.657, 48.5489) -> (8.1862, 48.8184) centre (0, 0) ccw projected
  arc A225 (8.1862, 48.8184) -> (7.3179, 53.5019) centre (-15.9886, 46.7583) ccw projected
  arc A226 (7.3179, 53.5019) -> (5.6986, 53.6985) centre (0, 0) ccw projected
  arc A227 (5.6986, 53.6985) -> (3.7346, 49.3589) centre (26.7139, 41.5733) ccw projected
  arc A228 (3.7346, 49.3589) -> (2.2421, 49.4492) centre (0, 0) ccw projected
  arc A229 (2.2421, 49.4492) -> (0.8156, 53.9938) centre (-21.5081, 44.4902) ccw projected
  arc A230 (0.8156, 53.9938) -> (-0.8156, 53.9938) centre (0, 0) ccw projected
  arc A231 (-0.8156, 53.9938) -> (-2.2421, 49.4492) centre (21.5081, 44.4902) ccw projected
  arc A232 (-2.2421, 49.4492) -> (-3.7346, 49.3589) centre (0, 0) ccw projected
  arc A233 (-3.7346, 49.3589) -> (-5.6986, 53.6985) centre (-26.7139, 41.5733) ccw projected
  arc A234 (-5.6986, 53.6985) -> (-7.3179, 53.5019) centre (0, 0) ccw projected
equation "\"d0\" = da_da"
equation "\"d1\" = da_b"
equation "\"d3\" = da_d"
equation "\"d16\" = da_aw"
equation "\"d43\" = da_aw"
equation "\"d46\" = da_aw"
equation "\"da_da\" = 108"
equation "\"da_b\" = 5"
equation "\"da_d\" = 104"
equation "\"da_aw\" = 65"
body "Solid1"
body "Srf1"
